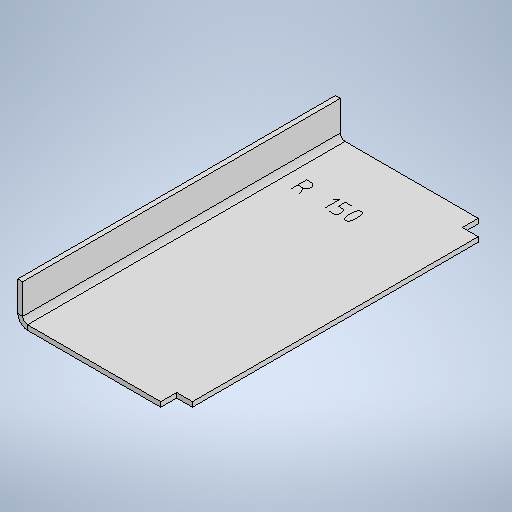
# Autodesk Inventor part: Part15
Saved by Autodesk Inventor 2025.3 (Build 293356030, 356C)
## iProperties
Created: 2026-01-14
Part Number: Part15
Material: Generic
Document SubType Name: Sheet Metal
Designer: admin
Density: 1 g/cm^3
Flat Pattern Width: 11.9702 cm
Flat Pattern Length: 20 cm
Flat Pattern Area: 239.405 cm^2
Sheet Metal Rule: Default
Sheet Metal Width: 119,702 mm
Sheet Metal Length: 200,000 mm
Sheet Metal Area: 23940,483 mm^2
Appearance: Default
Author: admin
Autodesk Inventor part; units mm, degrees
ref_plane "YZ Plane" through (0, 0, 0) normal (1, 0, 0) x (0, 1, 0)
ref_plane "XZ Plane" through (0, 0, 0) normal (0, 1, 0) x (-1, 0, 0)
ref_plane "XY Plane" through (0, 0, 0) normal (0, 0, 1) x (1, 0, 0)
sketch "Sketch1" plane through (0, 0, 0) normal (0, 0, 1) x (1, 0, 0)
  line L0 (0, 0) -> (100, 0)
  line L1 (100, 0) -> (100, -200)
  line L2 (100, -200) -> (0, -200)
  line L3 (0, -200) -> (0, 0)
  line L4 (100, 0) -> (90, 0)
  line L5 (90, 0) -> (90, -10)
  line L6 (90, -10) -> (100, -10)
  line L7 (100, -10) -> (100, 0)
  line L8 (100, -200) -> (90, -200)
  line L9 (90, -200) -> (90, -190)
  line L10 (90, -190) -> (100, -190)
  line L11 (100, -190) -> (100, -200)
  dimension "d0" = 100
  dimension "d1" = 200
  dimension "d2" = 10
  dimension "d3" = 10
  measures "d0" distance of L1.end L2.end
  measures "d1" distance of L0.end L1.end
  measures "d2" distance of L6.end L5.end
  measures "d3" distance of L5.end L4.end
extrude "Plate1" add sketch "Sketch1" along normal blind 3.048 contours L0 L5 L6 L1 L10 L9 L2 L3
sketch "Sketch2" plane through (0, 0, 3.048) normal (0, 0, 1) x (1, 0, 0)
  line L0 (13.9517, -33.0603) -> (49.292, -33.0603) construction
  line L1 (49.292, -33.0603) -> (49.292, -43.4735) construction
  line L2 (49.292, -43.4735) -> (13.9517, -43.4735) construction
  line L3 (13.9517, -43.4735) -> (13.9517, -33.0603) construction
  point P0 (0, 0)
  constraints: 2 other
mark "Mark1"
sketch "Sketch3" plane through (3.048, -200, 0) normal (-1, 0, 0) x (0, -1, 0)
  line L0 (-200, 0) -> (0, 0)
  line L1 (0, 0) -> (0, 25)
  line L2 (0, 25) -> (-200, 25)
  line L3 (-200, 25) -> (-200, 0)
  constraints: 6 end point, 1 horizontal, 1 perpendicular, 1 vertical
edge flange "Flange1" height 25 angle 90 thickness 3.048 bend radius 3.048 thickness toward (-1, 0, 0) relief tear relief width 3.048 relief depth 1.524 edges at (0, -100, 3.048) wall of the first edge with corners at (3.048, 0, 0) (3.048, -200, 0) (3.048, -200, 25) (3.048, 0, 25)
bend "Bend1"
corner "Corner1"
equation "\"d4\" = Thickness"
equation "\"d5\" = BendReliefWidth"
equation "\"d6\" = BendReliefDepth"
equation "\"d7\" = MinimumRemnant"
equation "\"d8\" = TransitionRadius"
equation "\"d11\" = BendRadius"
equation "\"d12\" = CornerReliefSize"
equation "\"d13\" = GapSize"
equation "\"d14\" = JacobiRadiusSize"
equation "\"BendRadius\" = Thickness"
equation "\"BendReliefWidth\" = Thickness"
equation "\"BendReliefDepth\" = 0.5 * Thickness"
equation "\"CornerReliefSize\" = 4 * Thickness"
equation "\"MinimumRemnant\" = 2 * Thickness"
equation "\"TransitionRadius\" = BendRadius"
equation "\"JacobiRadiusSize\" = BendRadius"
equation "\"GapSize\" = Thickness"
equation "\"Thickness\" = 3.048"
body "Solid1"
